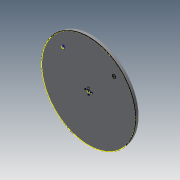
# Autodesk Inventor part: mainpulley
Saved by Autodesk Inventor 2015 (Build 190159000, 159)
## iProperties
Created: 2014-08-31
Part Number: mainpulley
Material: Generic
Document SubType Name: Modeling
Designer: shohei
Density: 1 g/cm^3
Appearance: Default
Mass: 1410.58 g
Surface Area: 1611.64 cm^2
Volume: 1410.58 cm^3
Author: shohei
Autodesk Inventor part; units mm, degrees
ref_plane "YZ Plane" through (0, 0, 0) normal (1, 0, 0) x (0, 1, 0)
ref_plane "XZ Plane" through (0, 0, 0) normal (0, 1, 0) x (-1, 0, 0)
ref_plane "XY Plane" through (0, 0, 0) normal (0, 0, 1) x (1, 0, 0)
sketch "Block1" plane through (0, 0, 0) normal (0, 0, 1) x (1, 0, 0)
  circle A0 centre (0, 0) radius 150.22
  circle A1 centre (0, 0) radius 5.22
  circle A2 centre (-0.0076, 30) radius 2.22
  circle A3 centre (30, 0.0076) radius 2.22
  circle A4 centre (0.0076, -30) radius 2.22
  circle A5 centre (-30, -0.0076) radius 2.22
  circle A6 centre (-81.3173, -81.3173) radius 5.22
  point P0 (-11.6168, -11.6168)
sketch "Block2" plane through (0, 0, 0) normal (0, 0, 1) x (1, 0, 0)
  circle A0 centre (0, 0) radius 150.22
  circle A1 centre (-81.3173, 81.3173) radius 5.22
  circle A2 centre (0, 10) radius 2.22
  circle A3 centre (-10, 0) radius 2.22
  circle A4 centre (0, 0) radius 5.22
  circle A5 centre (10, 0) radius 2.22
  circle A6 centre (0, -10) radius 2.22
  point P0 (-11.6168, 11.6168)
sketch "Sketch1" plane through (0, 0, 0) normal (0, 1, 0) x (-1, 0, 0)
  circle A0 centre (0, 0) radius 150
  circle A1 centre (0, 0) radius 5
  circle A2 centre (81.3173, 81.3173) radius 5
  line L0 (210.308, 0) -> (-210.308, 0) projected
  line L1 (0, -210.308) -> (0, 210.308) projected
  circle A3 centre (0, 10) radius 2
  circle A4 centre (-10, 0) radius 2
  circle A5 centre (0, -10) radius 2
  circle A6 centre (10, 0) radius 2
  dimension "d12" = 360
  dimension "d0" = 300
  dimension "d1" = 10
  dimension "d2" = 10
  dimension "d7" = 105
  dimension "d9" = 4
  dimension "d18" = 10
  constraints: 7 centre point, 3 coincident, 1 point on line, 9 other
  measures "d0" diameter of A0
  measures "d1" diameter of A1
  measures "d2" diameter of A2
  measures "d9" diameter of A3
  measures "d18" distance of A6.centre A1.centre
ref_plane "Work Plane1" through (0, 10, 0) normal (0, 1, 0) x (1, 0, 0)
extrude "Extrusion4" add sketch "Sketch1" along normal blind 10 contours L0 A6 A1 L1 A3 A0 | A0 L1 A5 A1 L0 A6 | L1 A3 A1 L0 A4 A0 | A0 L0 A4 A1 L1 A5
sketch "Sketch4" plane through (0, 0, 0) normal (0, -1, 0) x (1, 0, 0)
  circle A0 centre (-81.3173, 81.3173) radius 5 projected
  circle A1 centre (0, 0) radius 5 projected
  circle A2 centre (-10, 0) radius 2 projected
  circle A3 centre (0, -10) radius 2 projected
  circle A4 centre (10, 0) radius 2 projected
  circle A5 centre (0, 10) radius 2 projected
  circle A6 centre (0, 0) radius 150 projected
  constraints: 7 other
sketch "DXF" plane through (0, 0, 0) normal (0, 1, 0) x (-1, 0, 0)
  point P0 (0, 0)
equation "\"d0\" = pD"
equation "\"d7\" = 0.35 * pD"
equation "\"pD\" = 300"
body "Solid4"
